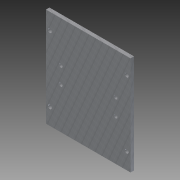
# Autodesk Inventor part: xy axis mount
Saved by Autodesk Inventor 2011 (Build 150239000, 239)
## iProperties
Created: 2013-10-30
Part Number: xy axis mount
Document SubType Name: Modeling
Designer: Devon
Density: 1 g/cm^3
Author: Devon
Autodesk Inventor part; units mm, degrees
ref_plane "YZ Plane" through (0, 0, 0) normal (1, 0, 0) x (0, 1, 0)
ref_plane "XZ Plane" through (0, 0, 0) normal (0, 1, 0) x (-1, 0, 0)
ref_plane "XY Plane" through (0, 0, 0) normal (0, 0, 1) x (1, 0, 0)
sketch "Sketch1" plane through (0, 0, 0) normal (0, 0, 1) x (1, 0, 0)
  line L0 (-43.0288, 68.3746) -> (111.0984, 68.3746)
  line L1 (111.0984, 68.3746) -> (111.0984, -111.7622)
  line L2 (111.0984, -111.7622) -> (-43.0288, -111.7622)
  line L3 (-43.0288, -111.7622) -> (-43.0288, 68.3746)
  line L4 (111.0984, 68.3746) -> (111.0984, 28.3696)
  line L5 (-43.0288, 68.3746) -> (-36.0288, 68.3746)
  line L6 (111.0984, 68.3746) -> (104.0984, 68.3746)
  line L7 (111.0984, -111.7622) -> (111.0984, -71.7572)
  line L8 (111.0984, 68.3746) -> (111.0984, 38.3746)
  line L9 (111.0984, -111.7622) -> (111.0984, -81.7622)
  circle A0 centre (104.0984, 38.3746) radius 3.5
  circle A1 centre (104.0984, -81.7622) radius 3.5
  circle A2 centre (-36.0288, 38.3746) radius 3.5
  circle A3 centre (-36.0288, -81.7622) radius 3.5
  circle A4 centre (-15.9652, -6.6938) radius 3.175
  circle A5 centre (-15.9652, -36.6938) radius 3.175
  circle A6 centre (84.0348, -36.6938) radius 3.175
  circle A7 centre (84.0348, -6.6938) radius 3.175
  point P0 (0, 0)
  dimension "d0" = 154.1272
  dimension "d1" = 180.1368
  dimension "d3" = 7
  dimension "d4" = 7
  dimension "d30" = 30
  dimension "d31" = 30
  dimension "d32" = 7
  dimension "d33" = 7
  dimension "d38" = 6.35
  dimension "d39" = 6.35
  dimension "d40" = 6.35
  dimension "d41" = 6.35
  constraints: 20 end point, 8 centre point, 6 point on line, 2 parallel, 1 horizontal, 1 perpendicular
  measures "d0" distance of L1.end L2.end
  measures "d1" distance of L0.end L1.end
  measures "d3" distance of L0.start L5.end
  measures "d4" distance of L0.end L6.end
  measures "d30" distance of L0.end L8.end
  measures "d31" distance of L1.end L9.end
  measures "d32" diameter of A0
  measures "d33" diameter of A1
  measures "d38" diameter of A4
  measures "d39" diameter of A5
  measures "d40" diameter of A6
  measures "d41" diameter of A7
extrude "Extrusion1" add sketch "Sketch1" along normal blind 6.35
body "Solid1"
